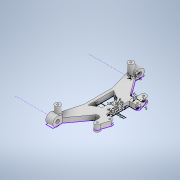
# Autodesk Inventor part: PX9200-11
Saved by Autodesk Inventor 2022.3 (Build 263350000, 350)
## iProperties
Created: 2022-07-21
Part Number: PX9200-11
Material: Generic
Document SubType Name: Modeling
Designer: luis_
Density: 1 g/cm^3
Appearance: Default
Author: luis_
Autodesk Inventor part; units mm, degrees
ref_plane "YZ Plane" through (0, 0, 0) normal (1, 0, 0) x (0, 1, 0)
ref_plane "XZ Plane" through (0, 0, 0) normal (0, 1, 0) x (-1, 0, 0)
ref_plane "XY Plane" through (0, 0, 0) normal (0, 0, 1) x (1, 0, 0)
sketch "Sketch1" plane through (0, 0, 0) normal (0, 1, 0) x (-1, 0, 0)
  line L0 (0, 0) -> (9, 0)
  line L1 (9, 0) -> (9, -12.5)
  line L2 (9, -12.5) -> (2.5, -12.5)
  circle A0 centre (2.5, -15) radius 2.5
  circle A1 centre (2.5, -15) radius 1
  line L3 (2.5, -15) -> (17.5, -15) construction
  circle A2 centre (6, -25.188) radius 3
  circle A3 centre (6, -25.188) radius 1
  line L4 (0, -15.4175) -> (3.0968, -24.4319)
  line L5 (9, 0) -> (17.3, 0)
  line L6 (17.3, 0) -> (17.3, -8)
  line L7 (17.3, -8) -> (27.3459, -13.8)
  line L8 (27.3459, -13.8) -> (27.3459, 0)
  line L9 (30.3459, 0) -> (30.3459, -15.6149)
  line L10 (30.3459, -15.6149) -> (37.3459, -39.6149)
  line L11 (37.3459, -39.6149) -> (37.3459, -49.6149)
  line L12 (29.6459, -39.6149) -> (29.6459, -49.6149)
  line L13 (37.3459, -49.6149) -> (29.6459, -49.6149)
  line L14 (29.6459, -39.6149) -> (80.5305, -39.6149) construction
  arc A4 (14.4139, -18.9731) -> (9, -20.7544) centre (12, -20.7544) ccw
  line L15 (29.6459, -39.6149) -> (19, -25.188)
  line L16 (19, -25.188) -> (16.5834, -21.9131)
  line L17 (16.5834, -21.9131) -> (14.4139, -18.9731)
  line L18 (9, -20.7544) -> (9, -25.188)
  circle A5 centre (12, -7) radius 1
  circle A6 centre (34.3459, -39.6149) radius 3
  circle A7 centre (34.3459, -39.6149) radius 1
  line L19 (30.3459, 0) -> (0, 0)
  line L20 (9, 0) -> (9, 12.5)
  line L21 (9, 12.5) -> (2.5, 12.5)
  circle A8 centre (2.5, 15) radius 2.5
  circle A9 centre (2.5, 15) radius 1
  line L22 (2.5, 15) -> (17.5, 15) construction
  circle A10 centre (6, 25.188) radius 3
  circle A11 centre (6, 25.188) radius 1
  line L23 (0, 15.4175) -> (3.0968, 24.4319)
  line L24 (17.3, 0) -> (17.3, 8)
  line L25 (17.3, 8) -> (27.3459, 13.8)
  line L26 (27.3459, 13.8) -> (27.3459, 0)
  line L27 (30.3459, 0) -> (30.3459, 15.6149)
  line L28 (30.3459, 15.6149) -> (37.3459, 39.6149)
  line L29 (37.3459, 39.6149) -> (37.3459, 49.6149)
  line L30 (29.6459, 39.6149) -> (29.6459, 49.6149)
  line L31 (37.3459, 49.6149) -> (29.6459, 49.6149)
  line L32 (29.6459, 39.6149) -> (80.5305, 39.6149) construction
  arc A12 (9, 20.7544) -> (14.4139, 18.9731) centre (12, 20.7544) ccw
  line L33 (29.6459, 39.6149) -> (19, 25.188)
  line L34 (19, 25.188) -> (16.5834, 21.9131)
  line L35 (16.5834, 21.9131) -> (14.4139, 18.9731)
  line L36 (9, 20.7544) -> (9, 25.188)
  circle A13 centre (12, 7) radius 1
  circle A14 centre (34.3459, 39.6149) radius 3
  circle A15 centre (34.3459, 39.6149) radius 1
  arc A16 (12, -9) -> (12, -5) centre (12, -7) ccw
  arc A17 (12, 5) -> (12, 9) centre (12, 7) ccw
  line L37 (12, 5) -> (9, 5)
  line L38 (12, 9) -> (9, 9)
  line L39 (12, -5) -> (9, -5)
  line L40 (12, -9) -> (9, -9)
  point P0 (0.1356, 15.8123)
  point P1 (0.1356, -15.8123)
  point P2 (36.8755, -38.0021)
  dimension "d3" = 5
  dimension "d0" = 9
  dimension "d1" = 12.5
  dimension "d4" = 2
  dimension "d7" = 6
  dimension "d9" = 2
  dimension "d13" = 8.3
  dimension "d14" = 8
  dimension "d15" = 11.6
  dimension "d16" = 120
  dimension "d17" = 3
  dimension "d20" = 7.7
  dimension "d21" = 10
  dimension "d23" = 6
  dimension "d24" = 10
  dimension "d27" = 2
  dimension "d28" = 7
  dimension "d29" = 6
  dimension "d30" = 2
  dimension "d31" = 4
  dimension "d32" = 4
  constraints: 82 end point, 26 symmetric about line, 16 centre point, 12 point on circle, 8 coincident, 7 horizontal, 6 perpendicular, 6 point on line, 6 tangent, 5 vertical, 1 collinear, 1 parallel, 15 other
  measures "d0" distance of L0.start L0.end
  measures "d1" distance of L0.end L1.end
  measures "d4" diameter of A1
  measures "d7" diameter of A2
  measures "d9" diameter of A3
  measures "d13" distance of L0.end L5.end
  measures "d14" distance of L5.end L6.end
  measures "d15" distance of L6.end L7.end
  measures "d16" angle of L7 L6
  measures "d17" distance between parallel lines of L8 L9
  measures "d20" distance of L10.end L12.start
  measures "d21" distance of L10.end L11.end
  measures "d23" diameter of A4
  measures "d24" distance of L18.end L15.end
  measures "d27" diameter of A5
  measures "d28" distance from line of L5 A5.centre
  measures "d29" diameter of A6
  measures "d30" diameter of A7
  measures "d31" diameter of A16
  measures "d32" diameter of A17
extrude "Extrusion1" add sketch "Sketch1" along normal blind 5 contours L5 L6 L7 L8 L19 L9 L10 A6 L11 L13 L12 L15 L16 L17 A4 L18 A2 L4 A0 L2 L1 L40 A16 L39 | L20 L37 A17 L38 L21 A8 L23 A10 L36 A12 L35 L34 L33 L30 L31 L29 A14 L28 L27 L19 L26 L25 L24 L5 | L39 A16 L40 L1 | L20 L38 A17 L37 | A0 | A8 | L10 A6 | A14 L28 | A2 | A10 picked at (36.5127, -38.9975) picked at (36.5127, 38.9975)
extrude "Extrusion2" cut sketch "Sketch1" along normal blind 2 contours L39 A16 L40 L1 | L20 L38 A17 L37 | A0 | A8
extrude "Extrusion3" add sketch "Sketch1" against normal blind 2 contours A2 | A10
sketch "Sketch2" plane through (0, 5, 0) normal (0, 1, 0) x (1, 0, 0)
  circle A0 centre (-34.3459, 39.6149) radius 1 projected
  line L0 (-37.3459, 49.6149) -> (-37.3459, 39.6149) projected
  circle A1 centre (-34.3459, 39.6149) radius 3
  circle A2 centre (-34.3459, -39.6149) radius 1 projected
  circle A3 centre (-34.3459, -39.6149) radius 3
  line L1 (-37.3459, -39.6149) -> (-37.3459, -49.6149) projected
  line L2 (-37.3459, -39.6149) -> (-37.3459, -49.6149)
  line L3 (-37.3459, -49.6149) -> (-29.6459, -49.6149) projected
  line L4 (-37.3459, -49.6149) -> (-29.6459, -49.6149)
  line L5 (-29.6459, -49.6149) -> (-29.6459, -39.6149) projected
  line L6 (-29.6459, -49.6149) -> (-29.6459, -39.6149)
  line L7 (-29.6459, -39.6149) -> (-31.3459, -39.6149)
  line L8 (-37.3459, 39.6149) -> (-37.3459, 49.6149)
  line L9 (-37.3459, 49.6149) -> (-29.6459, 49.6149)
  line L10 (-29.6459, 49.6149) -> (-29.6459, 39.6149)
  line L11 (-29.6459, 39.6149) -> (-31.3459, 39.6149)
  point P0 (0, 0)
  constraints: 16 end point, 4 perpendicular, 3 point on circle, 2 centre point, 2 coincident, 2 collinear, 2 point on line, 1 tangent
extrude "Extrusion5" add sketch "Sketch2" along normal blind 10 contours A1 | A3
extrude "Extrusion6" add sketch "Sketch2" along normal blind 3 contours L9 L10 L11 A1 L0 | L7 L5 L3 L1 A3
sketch "Sketch3" plane through (-37.3459, 0, 39.6149) normal (-1, 0, 0) x (0, 0, 1)
  circle A0 centre (5, 4) radius 2
  line L0 (10, 0) -> (10, 8) projected
  arc A1 (2, 0) -> (2, 8) centre (5, 4) ccw
  circle A2 centre (-84.2298, 4) radius 2
  line L1 (-89.2298, 0) -> (-89.2298, 8) projected
  arc A3 (-81.2298, 8) -> (-81.2298, 0) centre (-84.2298, 4) ccw
  line L2 (-89.2298, 0) -> (-79.2298, 0) projected
  line L3 (-87.2298, 0) -> (-89.2298, 0)
  line L4 (-89.2298, 0) -> (-89.2298, 8) projected
  line L5 (-89.2298, 0) -> (-89.2298, 8)
  line L6 (-89.2298, 8) -> (-87.2298, 8)
  line L7 (-79.2298, 8) -> (-89.2298, 8) projected
  arc A4 (-87.2298, 8) -> (-87.2298, 0) centre (-84.2298, 4) ccw
  line L8 (0, 0) -> (10, 0) projected
  line L9 (10, 8) -> (0, 8) projected
  arc A5 (8, 0) -> (8, 8) centre (5, 4) ccw
  line L10 (8, 0) -> (10, 0)
  line L11 (10, 8) -> (8, 8)
  point P0 (-39.6149, 0)
  point P1 (10, 4)
  point P2 (-89.2298, 4)
  dimension "d45" = 4
  dimension "d46" = 5
  dimension "d47" = 4
  dimension "d48" = 5
  constraints: 14 point on circle, 10 end point, 8 point on line, 6 centre point, 3 collinear, 2 coincident, 1 midpoint, 1 parallel
  measures "d45" diameter of A0
  measures "d46" distance of point (10, 4) A0.centre
  measures "d47" diameter of A2
  measures "d48" distance from line of L1 A2.centre
extrude "Extrusion7" add sketch "Sketch3" against normal blind 7.7 contours A1 L8 | L9 A1 | A3 L7 | L2 A3
extrude "Extrusion8" cut sketch "Sketch3" against normal blind 10 contours A0 | L8 A1 L0 | A1 L9 L0 | A2 | L1 L6 A3 | L1 A3 L2
body "Solid1"
